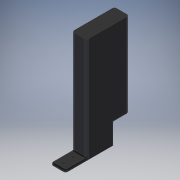
# Autodesk Inventor part: ButtonMountLegs
Saved by Autodesk Inventor 2018 (Build 220112000, 112)
## iProperties
Created: 2018-05-19
Part Number: ButtonMountLegs
Material: Generic
Document SubType Name: Modeling
Designer: reide
Density: 1 g/cm^3
Appearance: Default
Author: reide
Autodesk Inventor part; units mm, degrees
(part 1 of 2)
ref_plane "YZ Plane" through (0, 0, 0) normal (1, 0, 0) x (0, 1, 0)
sketch "Sketch1" plane through (0, 0, 0) normal (0, 0, 1) x (1, 0, 0)
  circle A0 centre (68.6105, -28.321) radius 1.63 projected
  arc A1 (92.5111, 275.0837) -> (88.5111, 275.0837) centre (90.5111, 275.0837) ccw projected
  line L0 (92.5111, 275.0837) -> (92.5111, 230.0837) projected
  arc A2 (88.5111, 230.0837) -> (92.5111, 230.0837) centre (90.5111, 230.0837) ccw projected
  line L1 (88.5111, 230.0837) -> (88.5111, 275.0837) projected
  arc A3 (47.5111, 275.0837) -> (43.5111, 275.0837) centre (45.5111, 275.0837) ccw projected
  line L2 (47.5111, 275.0837) -> (47.5111, 230.0837) projected
  arc A4 (43.5111, 230.0837) -> (47.5111, 230.0837) centre (45.5111, 230.0837) ccw projected
  line L3 (43.5111, 230.0837) -> (43.5111, 275.0837) projected
  circle A5 centre (6.132, -79.3472) radius 1.25 projected
  circle A6 centre (145.3842, 185.8247) radius 1.5 projected
  circle A7 centre (153.8932, -1.3222) radius 1.5 projected
  circle A8 centre (145.3842, -79.3472) radius 1.5 projected
  circle A9 centre (129.8902, 6.8528) radius 1.5 projected
  circle A10 centre (116.3012, -71.1722) radius 1.5 projected
  circle A11 centre (129.8902, 272.0247) radius 1.5 projected
  circle A12 centre (129.8902, 185.8247) radius 1.5 projected
  circle A13 centre (116.3012, 263.8497) radius 1.5 projected
  circle A14 centre (-17.871, -71.1722) radius 1.5 projected
  circle A15 centre (6.132, 6.8528) radius 1.5 projected
  circle A16 centre (19.721, -1.3222) radius 1.5 projected
  circle A17 centre (-17.871, 263.8497) radius 1.5 projected
  circle A18 centre (-9.362, 272.0247) radius 1.5 projected
  circle A19 centre (-9.362, 185.8247) radius 1.5 projected
  circle A20 centre (19.721, 193.9997) radius 1.5 projected
  circle A21 centre (19.721, 263.8497) radius 1.5 projected
  circle A22 centre (6.132, 185.8247) radius 1.5 projected
  circle A23 centre (6.132, 272.0247) radius 1.5 projected
  circle A24 centre (-17.871, 193.9997) radius 1.5 projected
  circle A25 centre (19.721, -71.1722) radius 1.5 projected
  circle A26 centre (-9.362, -79.3472) radius 1.5 projected
  circle A27 centre (-9.362, 6.8528) radius 1.5 projected
  circle A28 centre (-17.871, -1.3222) radius 1.5 projected
  circle A29 centre (116.3012, 193.9997) radius 1.5 projected
  circle A30 centre (153.8932, 193.9997) radius 1.5 projected
  circle A31 centre (153.8932, 263.8497) radius 1.5 projected
  circle A32 centre (145.3842, 6.8528) radius 1.5 projected
  circle A33 centre (129.8902, -79.3472) radius 1.5 projected
  circle A34 centre (153.8932, -71.1722) radius 1.5 projected
  circle A35 centre (116.3012, -1.3222) radius 1.5 projected
  circle A36 centre (145.3842, 272.0247) radius 1.5 projected
  arc A37 (-56.4499, 266.1206) -> (-81.2372, 206.8201) centre (44.5185, 189.0856) ccw projected
  arc A38 (-81.2372, 206.8201) -> (-81.2372, -14.1426) centre (702.1899, 96.3387) ccw projected
  arc A39 (-81.2372, -14.1426) -> (-56.4499, -73.4431) centre (44.5185, 3.5918) ccw projected
  ellipse E0 centre (68.0111, 96.3387) end of major axis (68.0111, -141.4053) minor radius 177.8 (-56.4499, -73.4431) -> (192.4721, -73.4431) ccw projected
  arc A40 (192.4721, -73.4431) -> (217.2594, -14.1426) centre (91.5037, 3.5918) ccw projected
  arc A41 (217.2594, -14.1426) -> (217.2594, 206.8201) centre (-566.1677, 96.3387) ccw projected
  arc A42 (217.2594, 206.8201) -> (192.4721, 266.1206) centre (91.5037, 189.0856) ccw projected
  ellipse E1 centre (68.0111, 96.3387) end of major axis (68.0111, -141.4053) minor radius 177.8 (192.4721, 266.1206) -> (-56.4499, 266.1206) ccw projected
  line L4 (127.3658, 171.3576) -> (131.3658, 171.3576) projected
  arc A43 (131.3658, 168.3578) -> (131.3658, 171.3576) centre (131.3658, 169.8577) ccw projected
  line L5 (131.3658, 168.3578) -> (127.3658, 168.3578) projected
  arc A44 (127.3658, 171.3576) -> (127.3658, 168.3578) centre (127.3658, 169.8577) ccw projected
  line L6 (127.3198, 106.6744) -> (131.3198, 106.6744) projected
  arc A45 (131.3198, 103.6746) -> (131.3198, 106.6744) centre (131.3198, 105.1745) ccw projected
  line L7 (131.3198, 103.6746) -> (127.3198, 103.6746) projected
  arc A46 (127.3198, 106.6744) -> (127.3198, 103.6746) centre (127.3198, 105.1745) ccw projected
  line L8 (12.8629, 171.439) -> (16.8629, 171.439) projected
  arc A47 (16.8629, 168.4391) -> (16.8629, 171.439) centre (16.8629, 169.9391) ccw projected
  line L9 (16.8629, 168.4391) -> (12.8629, 168.4391) projected
  arc A48 (12.8629, 171.439) -> (12.8629, 168.4391) centre (12.8629, 169.9391) ccw projected
  line L10 (12.8169, 106.6744) -> (16.8169, 106.6744) projected
  arc A49 (16.8169, 103.6746) -> (16.8169, 106.6744) centre (16.8169, 105.1745) ccw projected
  line L11 (16.8169, 103.6746) -> (12.8169, 103.6746) projected
  arc A50 (12.8169, 106.6744) -> (12.8169, 103.6746) centre (12.8169, 105.1745) ccw projected
  arc A51 (101.8543, 86.6033) -> (98.8567, 86.6032) centre (100.3555, 86.6032) ccw projected
  line L12 (101.8543, 86.6033) -> (101.8544, 82.6033) projected
  arc A52 (98.8565, 82.6033) -> (101.8544, 82.6033) centre (100.3555, 82.6032) ccw projected
  line L13 (98.8565, 82.6033) -> (98.8567, 86.6032) projected
  arc A53 (101.9362, 200.9947) -> (98.9379, 201.0395) centre (100.4367, 200.9934) ccw projected
  line L14 (101.9362, 200.9947) -> (101.9357, 196.9932) projected
  arc A54 (98.9377, 196.9935) -> (101.9357, 196.9932) centre (100.4367, 196.9934) ccw projected
  line L15 (98.9377, 196.9935) -> (98.9379, 201.0395) projected
  line L16 (34.0863, 189.3896) -> (34.0865, 193.3895) projected
  arc A55 (37.0841, 193.3896) -> (34.0865, 193.3895) centre (35.5853, 193.3895) ccw projected
  line L17 (37.0841, 193.3896) -> (37.0843, 189.3896) projected
  arc A56 (34.0863, 189.3896) -> (37.0843, 189.3896) centre (35.5853, 189.3895) ccw projected
  arc A57 (101.8488, 78.9533) -> (98.8512, 78.9533) centre (100.35, 78.9533) ccw projected
  line L18 (101.8488, 78.9533) -> (101.849, 74.9533) projected
  arc A58 (98.851, 74.9533) -> (101.849, 74.9533) centre (100.35, 74.9533) ccw projected
  line L19 (98.851, 74.9533) -> (98.8512, 78.9533) projected
  circle A59 centre (95.163, 40.4375) radius 1.25 projected
  circle A60 centre (46.141, 40.2217) radius 1.25 projected
  circle A61 centre (36.616, 12.9421) radius 1.25 projected
  circle A62 centre (36.616, -11.1741) radius 1.25 projected
  circle A63 centre (46.141, -14.3491) radius 1.25 projected
  circle A64 centre (36.616, 37.0467) radius 1.25 projected
  circle A65 centre (95.163, -4.4165) radius 1.25 projected
  arc A66 (101.9301, 193.3866) -> (98.9325, 193.3865) centre (100.4313, 193.3865) ccw projected
  line L20 (101.9301, 193.3866) -> (101.9303, 189.3866) projected
  arc A67 (98.9323, 189.3866) -> (101.9303, 189.3866) centre (100.4313, 189.3865) ccw projected
  line L21 (98.9323, 189.3866) -> (98.9325, 193.3865) projected
  arc A68 (37.0788, 78.9992) -> (34.0812, 78.9993) centre (35.58, 78.9992) ccw projected
  line L22 (37.0788, 78.9992) -> (37.079, 74.9993) projected
  arc A69 (34.081, 74.9993) -> (37.079, 74.9993) centre (35.58, 74.9992) ccw projected
  line L23 (34.081, 74.9993) -> (34.0812, 78.9993) projected
  arc A70 (37.0841, 201.0395) -> (34.0865, 201.0395) centre (35.5853, 201.0395) ccw projected
  line L24 (37.0841, 201.0395) -> (37.0843, 197.0395) projected
  arc A71 (34.0863, 197.0396) -> (37.0843, 197.0395) centre (35.5853, 197.0395) ccw projected
  line L25 (34.0863, 197.0396) -> (34.0865, 201.0395) projected
  arc A72 (37.0792, 86.6494) -> (34.0816, 86.6493) centre (35.5804, 86.6492) ccw projected
  line L26 (37.0792, 86.6494) -> (37.0794, 82.6493) projected
  arc A73 (34.0814, 82.6493) -> (37.0794, 82.6493) centre (35.5804, 82.6492) ccw projected
  line L27 (34.0814, 82.6493) -> (34.0816, 86.6493) projected
  line L28 (9.1669, 103.6742) -> (5.1669, 103.6742) projected
  arc A74 (5.1669, 106.6741) -> (5.1669, 103.6742) centre (5.1669, 105.1742) ccw projected
  line L29 (5.1669, 106.6741) -> (9.1669, 106.6741) projected
  arc A75 (9.1669, 103.6742) -> (9.1669, 106.6741) centre (9.1669, 105.1742) ccw projected
  line L30 (5.1669, 171.4444) -> (9.1669, 171.4444) projected
  arc A76 (9.1669, 168.4446) -> (9.1669, 171.4444) centre (9.1669, 169.9445) ccw projected
  line L31 (9.1669, 168.4446) -> (5.1669, 168.4446) projected
  arc A77 (5.1669, 171.4444) -> (5.1669, 168.4446) centre (5.1669, 169.9445) ccw projected
  line L32 (119.6698, 106.6744) -> (123.6698, 106.6744) projected
  arc A78 (123.6698, 103.6746) -> (123.6698, 106.6744) centre (123.6698, 105.1745) ccw projected
  line L33 (123.6698, 103.6746) -> (119.6698, 103.6746) projected
  arc A79 (119.6698, 106.6744) -> (119.6698, 103.6746) centre (119.6698, 105.1745) ccw projected
  line L34 (119.7158, 171.3631) -> (123.7158, 171.3631) projected
  arc A80 (123.7158, 168.3632) -> (123.7158, 171.3631) centre (123.7158, 169.8631) ccw projected
  line L35 (123.7158, 168.3632) -> (119.7158, 168.3632) projected
  arc A81 (119.7158, 171.3631) -> (119.7158, 168.3632) centre (119.7158, 169.8631) ccw projected
  circle A82 centre (68.0111, 137.616) radius 35 projected
  line L36 (82.971, 43.3967) -> (82.971, -17.5241) projected
  line L37 (82.971, -17.5241) -> (52.491, -17.5241) projected
  line L38 (52.491, -17.5241) -> (52.491, 43.3967) projected
  line L39 (52.491, 43.3967) -> (82.971, 43.3967) projected
  circle A83 centre (56.9111, -110.4053) radius 1.5 projected
  circle A84 centre (79.1111, -110.4053) radius 1.5 projected
  circle A85 centre (77.2861, -128.5803) radius 1.5 projected
  circle A86 centre (85.0931, -46.904) radius 1.5 projected
  circle A87 centre (92.2681, -54.079) radius 1.5 projected
  circle A88 centre (53.9141, -54.079) radius 1.5 projected
  circle A89 centre (61.0891, -46.904) radius 1.5 projected
  circle A90 centre (58.7361, -128.5803) radius 1.5 projected
  circle A91 centre (79.1111, -118.4053) radius 1.5 projected
  circle A92 centre (56.9111, -118.4053) radius 1.5 projected
  circle A93 centre (35.6216, 318.7587) radius 1.25 projected
  circle A94 centre (100.4006, 248.9087) radius 1.25 projected
  circle A95 centre (100.4006, 318.7587) radius 1.25 projected
  circle A96 centre (35.6216, 248.9087) radius 1.25 projected
  line L40 (68.0111, 137.616) -> (68.0111, -141.4053)
  line L41 (68.0111, -141.4053) -> (68.0111, 334.0827)
  line L42 (68.0111, 96.3387) -> (-88.9891, 96.3387)
  line L43 (16.9653, 102.9185) -> (4.9653, 102.9185) projected
  arc A97 (4.9653, 118.4285) -> (3.9653, 117.4285) centre (4.9653, 117.4285) ccw projected
  line L44 (4.9653, 118.4285) -> (16.9653, 118.4285) projected
  arc A98 (17.9653, 117.4285) -> (16.9653, 118.4285) centre (16.9653, 117.4285) ccw projected
  line L45 (17.9653, 117.4285) -> (17.9653, 102.9185) projected
  arc A99 (16.9653, 101.9185) -> (17.9653, 102.9185) centre (16.9653, 102.9185) ccw projected
  line L46 (16.9653, 101.9185) -> (4.9653, 101.9185) projected
  arc A100 (3.9653, 102.9185) -> (4.9653, 101.9185) centre (4.9653, 102.9185) ccw projected
  line L47 (3.9653, 117.4285) -> (3.9653, 102.9185) projected
  circle A101 centre (7.1403, 105.0935) radius 1.5 projected
  circle A102 centre (14.7903, 105.0935) radius 1.5 projected
  line L48 (17.6724, 96.3387) -> (3.9653, 96.3387)
  line L49 (3.9653, 96.3387) -> (3.9653, 101.9185)
  line L50 (3.9653, 101.9185) -> (17.6724, 101.9185)
  line L51 (17.6724, 101.9185) -> (17.6724, 96.3387)
  line L52 (17.6724, 96.3387) -> (3.9653, 96.3387)
  line L53 (3.9653, 96.3387) -> (3.9653, 56.3387)
  line L54 (3.9653, 56.3387) -> (17.6724, 56.3387)
  line L55 (17.6724, 56.3387) -> (17.6724, 96.3387)
  circle A103 centre (125.2036, 96.9184) radius 1.75 projected
  circle A104 centre (10.8185, 96.9184) radius 1.75 projected
  circle A105 centre (10.8187, 86.9184) radius 1.75 projected
  circle A106 centre (125.2035, 86.9184) radius 1.75 projected
  circle A107 centre (125.2039, 71.3387) radius 1.75 projected
  circle A108 centre (10.8188, 71.3387) radius 1.75 projected
  circle A109 centre (10.8188, 61.3387) radius 1.75 projected
  circle A110 centre (125.2039, 61.3387) radius 1.75 projected
  point P0 (0, 0)
  dimension "d0" = 40
  constraints: 22 end point, 4 parallel, 2 horizontal, 2 perpendicular, 1 point on circle, 1 point on line, 1 vertical, 4 other
  measures "d0" distance of L54.end L48.start
ref_plane "Work Plane1" through (4.9653, 102.9185, 2) normal (0, 0, 1) x (1, 0, 0)
extrude "Extrusion1" add sketch "Sketch1" along normal up to surface (2 mm away) contours L55 L54 L53 L42 A104 | L42 A104 L49 L50 L46 L51 | A104 L42 | L42 A104 | A105 | A108 | A109
sketch "Sketch2" plane through (3.9653, 101.9185, 2) normal (0, 0, 1) x (1, 0, 0)
  line L0 (13.7071, -45.5798) -> (13.7071, 0) projected
  line L1 (13.7071, -45.5798) -> (13.7071, 34.4202)
  line L2 (0, -45.5798) -> (13.7071, -45.5798) projected
  line L3 (0, -45.5798) -> (0, -5.5798)
  line L4 (0, 0) -> (0, -45.5798) projected
  line L5 (0, -5.5798) -> (0, -25.5798)
  line L6 (0, -25.5798) -> (13.7071, -25.5798)
  line L7 (13.7071, -25.5798) -> (0, -25.5798)
  line L8 (0, -25.5798) -> (0, 0)
  line L9 (0, 0) -> (13.7071, 0)
  line L10 (13.7071, 0) -> (13.7071, -25.5798)
  circle A0 centre (64.6452, -130.2395) radius 1.63 projected
  arc A1 (88.5458, 173.1652) -> (84.5458, 173.1652) centre (86.5458, 173.1652) ccw projected
  line L11 (88.5458, 173.1652) -> (88.5458, 128.1652) projected
  arc A2 (84.5458, 128.1652) -> (88.5458, 128.1652) centre (86.5458, 128.1652) ccw projected
  line L12 (84.5458, 128.1652) -> (84.5458, 173.1652) projected
  arc A3 (43.5458, 173.1652) -> (39.5458, 173.1652) centre (41.5458, 173.1652) ccw projected
  line L13 (43.5458, 173.1652) -> (43.5458, 128.1652) projected
  arc A4 (39.5458, 128.1652) -> (43.5458, 128.1652) centre (41.5458, 128.1652) ccw projected
  line L14 (39.5458, 128.1652) -> (39.5458, 173.1652) projected
  circle A5 centre (2.1667, -181.2657) radius 1.25 projected
  circle A6 centre (141.4189, 83.9062) radius 1.5 projected
  circle A7 centre (149.9279, -103.2407) radius 1.5 projected
  circle A8 centre (141.4189, -181.2657) radius 1.5 projected
  circle A9 centre (125.9249, -95.0657) radius 1.5 projected
  circle A10 centre (112.3359, -173.0907) radius 1.5 projected
  circle A11 centre (125.9249, 170.1062) radius 1.5 projected
  circle A12 centre (125.9249, 83.9062) radius 1.5 projected
  circle A13 centre (112.3359, 161.9312) radius 1.5 projected
  circle A14 centre (-21.8363, -173.0907) radius 1.5 projected
  circle A15 centre (2.1667, -95.0657) radius 1.5 projected
  circle A16 centre (15.7557, -103.2407) radius 1.5 projected
  circle A17 centre (-21.8363, 161.9312) radius 1.5 projected
  circle A18 centre (-13.3273, 170.1062) radius 1.5 projected
  circle A19 centre (-13.3273, 83.9062) radius 1.5 projected
  circle A20 centre (15.7557, 92.0812) radius 1.5 projected
  circle A21 centre (15.7557, 161.9312) radius 1.5 projected
  circle A22 centre (2.1667, 83.9062) radius 1.5 projected
  circle A23 centre (2.1667, 170.1062) radius 1.5 projected
  circle A24 centre (-21.8363, 92.0812) radius 1.5 projected
  circle A25 centre (15.7557, -173.0907) radius 1.5 projected
  circle A26 centre (-13.3273, -181.2657) radius 1.5 projected
  circle A27 centre (-13.3273, -95.0657) radius 1.5 projected
  circle A28 centre (-21.8363, -103.2407) radius 1.5 projected
  circle A29 centre (112.3359, 92.0812) radius 1.5 projected
  circle A30 centre (149.9279, 92.0812) radius 1.5 projected
  circle A31 centre (149.9279, 161.9312) radius 1.5 projected
  circle A32 centre (141.4189, -95.0657) radius 1.5 projected
  circle A33 centre (125.9249, -181.2657) radius 1.5 projected
  circle A34 centre (149.9279, -173.0907) radius 1.5 projected
  circle A35 centre (112.3359, -103.2407) radius 1.5 projected
  circle A36 centre (141.4189, 170.1062) radius 1.5 projected
  arc A37 (-60.4152, 164.2021) -> (-85.2025, 104.9016) centre (40.5532, 87.1671) ccw projected
  arc A38 (-85.2025, 104.9016) -> (-85.2025, -116.0611) centre (698.2246, -5.5798) ccw projected
  arc A39 (-85.2025, -116.0611) -> (-60.4152, -175.3616) centre (40.5532, -98.3267) ccw projected
  ellipse E0 centre (64.0458, -5.5798) end of major axis (64.0458, -243.3238) minor radius 177.8 (-60.4152, -175.3616) -> (188.5068, -175.3616) ccw projected
  arc A40 (188.5068, -175.3616) -> (213.2941, -116.0611) centre (87.5384, -98.3267) ccw projected
  arc A41 (213.2941, -116.0611) -> (213.2941, 104.9016) centre (-570.133, -5.5798) ccw projected
  arc A42 (213.2941, 104.9016) -> (188.5068, 164.2021) centre (87.5384, 87.1671) ccw projected
  ellipse E1 centre (64.0458, -5.5798) end of major axis (64.0458, -243.3238) minor radius 177.8 (188.5068, 164.2021) -> (-60.4152, 164.2021) ccw projected
  line L15 (123.4005, 69.4391) -> (127.4005, 69.4391) projected
  arc A43 (127.4005, 66.4393) -> (127.4005, 69.4391) centre (127.4005, 67.9392) ccw projected
  line L16 (127.4005, 66.4393) -> (123.4005, 66.4393) projected
  arc A44 (123.4005, 69.4391) -> (123.4005, 66.4393) centre (123.4005, 67.9392) ccw projected
  line L17 (123.3545, 4.7559) -> (127.3545, 4.7559) projected
  arc A45 (127.3545, 1.7561) -> (127.3545, 4.7559) centre (127.3545, 3.256) ccw projected
  line L18 (127.3545, 1.7561) -> (123.3545, 1.7561) projected
  arc A46 (123.3545, 4.7559) -> (123.3545, 1.7561) centre (123.3545, 3.256) ccw projected
  line L19 (8.8976, 69.5205) -> (12.8976, 69.5205) projected
  arc A47 (12.8976, 66.5206) -> (12.8976, 69.5205) centre (12.8976, 68.0206) ccw projected
  line L20 (12.8976, 66.5206) -> (8.8976, 66.5206) projected
  arc A48 (8.8976, 69.5205) -> (8.8976, 66.5206) centre (8.8976, 68.0206) ccw projected
  line L21 (8.8516, 4.7559) -> (12.8516, 4.7559) projected
  arc A49 (12.8516, 1.7561) -> (12.8516, 4.7559) centre (12.8516, 3.256) ccw projected
  line L22 (12.8516, 1.7561) -> (8.8516, 1.7561) projected
  arc A50 (8.8516, 4.7559) -> (8.8516, 1.7561) centre (8.8516, 3.256) ccw projected
  arc A51 (97.889, -15.3152) -> (94.8914, -15.3153) centre (96.3902, -15.3153) ccw projected
  line L23 (97.889, -15.3152) -> (97.8892, -19.3152) projected
  arc A52 (94.8912, -19.3152) -> (97.8892, -19.3152) centre (96.3902, -19.3153) ccw projected
  line L24 (94.8912, -19.3152) -> (94.8914, -15.3153) projected
  arc A53 (97.9709, 99.0762) -> (94.9726, 99.121) centre (96.4714, 99.0749) ccw projected
  line L25 (97.9709, 99.0762) -> (97.9704, 95.0747) projected
  arc A54 (94.9724, 95.075) -> (97.9704, 95.0747) centre (96.4714, 95.0749) ccw projected
  line L26 (94.9724, 95.075) -> (94.9726, 99.121) projected
  line L27 (30.121, 87.4711) -> (30.1212, 91.471) projected
  arc A55 (33.1188, 91.4711) -> (30.1212, 91.471) centre (31.62, 91.471) ccw projected
  line L28 (33.1188, 91.4711) -> (33.119, 87.4711) projected
  arc A56 (30.121, 87.4711) -> (33.119, 87.4711) centre (31.62, 87.471) ccw projected
  arc A57 (97.8835, -22.9652) -> (94.8859, -22.9652) centre (96.3847, -22.9652) ccw projected
  line L29 (97.8835, -22.9652) -> (97.8837, -26.9652) projected
  arc A58 (94.8858, -26.9652) -> (97.8837, -26.9652) centre (96.3847, -26.9652) ccw projected
  line L30 (94.8858, -26.9652) -> (94.8859, -22.9652) projected
  circle A59 centre (91.1977, -61.481) radius 1.25 projected
  circle A60 centre (42.1757, -61.6968) radius 1.25 projected
  circle A61 centre (32.6507, -88.9764) radius 1.25 projected
  circle A62 centre (32.6507, -113.0926) radius 1.25 projected
  circle A63 centre (42.1757, -116.2676) radius 1.25 projected
  circle A64 centre (32.6507, -64.8718) radius 1.25 projected
  circle A65 centre (91.1977, -106.335) radius 1.25 projected
  arc A66 (97.9648, 91.4681) -> (94.9672, 91.468) centre (96.466, 91.468) ccw projected
  line L31 (97.9648, 91.4681) -> (97.965, 87.4681) projected
  arc A67 (94.967, 87.4681) -> (97.965, 87.4681) centre (96.466, 87.468) ccw projected
  line L32 (94.967, 87.4681) -> (94.9672, 91.468) projected
  arc A68 (33.1136, -22.9193) -> (30.116, -22.9192) centre (31.6148, -22.9193) ccw projected
  line L33 (33.1136, -22.9193) -> (33.1137, -26.9192) projected
  arc A69 (30.1158, -26.9192) -> (33.1137, -26.9192) centre (31.6148, -26.9193) ccw projected
  line L34 (30.1158, -26.9192) -> (30.116, -22.9192) projected
  arc A70 (33.1188, 99.121) -> (30.1212, 99.121) centre (31.62, 99.121) ccw projected
  line L35 (33.1188, 99.121) -> (33.119, 95.121) projected
  arc A71 (30.121, 95.1211) -> (33.119, 95.121) centre (31.62, 95.121) ccw projected
  line L36 (30.121, 95.1211) -> (30.1212, 99.121) projected
  arc A72 (33.1139, -15.2691) -> (30.1163, -15.2692) centre (31.6151, -15.2693) ccw projected
  line L37 (33.1139, -15.2691) -> (33.1141, -19.2692) projected
  arc A73 (30.1161, -19.2692) -> (33.1141, -19.2692) centre (31.6151, -19.2693) ccw projected
  line L38 (30.1161, -19.2692) -> (30.1163, -15.2692) projected
  line L39 (5.2016, 1.7558) -> (1.2016, 1.7558) projected
  arc A74 (1.2016, 4.7556) -> (1.2016, 1.7558) centre (1.2016, 3.2557) ccw projected
  line L40 (1.2016, 4.7556) -> (5.2016, 4.7556) projected
  arc A75 (5.2016, 1.7558) -> (5.2016, 4.7556) centre (5.2016, 3.2557) ccw projected
  line L41 (1.2016, 69.5259) -> (5.2016, 69.5259) projected
  arc A76 (5.2016, 66.5261) -> (5.2016, 69.5259) centre (5.2016, 68.026) ccw projected
  line L42 (5.2016, 66.5261) -> (1.2016, 66.5261) projected
  arc A77 (1.2016, 69.5259) -> (1.2016, 66.5261) centre (1.2016, 68.026) ccw projected
  line L43 (115.7045, 4.7559) -> (119.7045, 4.7559) projected
  arc A78 (119.7045, 1.7561) -> (119.7045, 4.7559) centre (119.7045, 3.256) ccw projected
  line L44 (119.7045, 1.7561) -> (115.7045, 1.7561) projected
  arc A79 (115.7045, 4.7559) -> (115.7045, 1.7561) centre (115.7045, 3.256) ccw projected
  line L45 (115.7505, 69.4446) -> (119.7505, 69.4446) projected
  arc A80 (119.7505, 66.4447) -> (119.7505, 69.4446) centre (119.7505, 67.9446) ccw projected
  line L46 (119.7505, 66.4447) -> (115.7505, 66.4447) projected
  arc A81 (115.7505, 69.4446) -> (115.7505, 66.4447) centre (115.7505, 67.9446) ccw projected
  circle A82 centre (64.0458, 35.6975) radius 35 projected
  line L47 (79.0057, -58.5218) -> (79.0057, -119.4426) projected
  line L48 (79.0057, -119.4426) -> (48.5257, -119.4426) projected
  line L49 (48.5257, -119.4426) -> (48.5257, -58.5218) projected
  line L50 (48.5257, -58.5218) -> (79.0057, -58.5218) projected
  circle A83 centre (52.9458, -212.3238) radius 1.5 projected
  circle A84 centre (75.1458, -212.3238) radius 1.5 projected
  circle A85 centre (73.3208, -230.4988) radius 1.5 projected
  circle A86 centre (81.1278, -148.8225) radius 1.5 projected
  circle A87 centre (88.3028, -155.9975) radius 1.5 projected
  circle A88 centre (49.9488, -155.9975) radius 1.5 projected
  circle A89 centre (57.1238, -148.8225) radius 1.5 projected
  circle A90 centre (54.7708, -230.4988) radius 1.5 projected
  circle A91 centre (75.1458, -220.3238) radius 1.5 projected
  circle A92 centre (52.9458, -220.3238) radius 1.5 projected
  circle A93 centre (31.6563, 216.8402) radius 1.25 projected
  circle A94 centre (96.4353, 146.9902) radius 1.25 projected
  circle A95 centre (96.4353, 216.8402) radius 1.25 projected
  circle A96 centre (31.6563, 146.9902) radius 1.25 projected
  line L51 (64.0458, 35.6975) -> (64.0458, -5.5798)
  circle A97 centre (121.2384, -5.0001) radius 1.75 projected
  circle A98 centre (6.8533, -5.0001) radius 1.75 projected
  circle A99 centre (6.8534, -15.0001) radius 1.75 projected
  circle A100 centre (121.2382, -15.0001) radius 1.75 projected
  circle A101 centre (121.2387, -30.5798) radius 1.75 projected
  circle A102 centre (6.8536, -30.5798) radius 1.75 projected
  circle A103 centre (6.8536, -40.5798) radius 1.75 projected
  circle A104 centre (121.2387, -40.5798) radius 1.75 projected
  point P0 (-3.9653, -101.9185)
  dimension "d3" = 80
  dimension "d4" = 40
  dimension "d5" = 20
  constraints: 18 end point, 3 point on line, 2 parallel, 2 perpendicular, 1 collinear, 1 horizontal, 1 vertical, 2 other
  measures "d3" distance of L0.start L1.end
  measures "d4" distance of L2.start L3.end
  measures "d5" distance of L3.end L5.end
ref_plane "Work Plane2" through (4.9653, 109.2685, 19.05) normal (0, 0, 1) x (1, 0, 0)
extrude "Extrusion2" add sketch "Sketch2" along normal up to surface (17.05 mm away) contours L6 L3 L4 L9 L0 | A98 | A99
sketch "Sketch3" plane through (3.9653, 101.9185, 19.05) normal (0, 0, 1) x (1, 0, 0)
  line L0 (0, -45.5798) -> (0, -25.5798) projected
  line L1 (13.7071, -45.5798) -> (0, -45.5798) projected
  line L2 (13.7071, -25.5798) -> (13.7071, -45.5798) projected
  line L3 (0, 0) -> (13.7071, 0) projected
  line L4 (0, -25.5798) -> (0, 0) projected
  line L5 (13.7071, -25.5798) -> (0, -25.5798) projected
  line L6 (13.7071, 0) -> (13.7071, -25.5798) projected
  line L7 (0, -45.5798) -> (13.7071, -45.5798) projected
  line L8 (0, -45.5798) -> (-80, -45.5798)
  line L9 (0, 0) -> (0, -45.5798) projected
  line L10 (0, -45.5798) -> (0, 34.4202)
  line L11 (13.7071, -45.5798) -> (13.7071, -5.5798)
  line L12 (13.7071, -45.5798) -> (13.7071, 0) projected
  line L13 (13.7071, -5.5798) -> (13.7071, 14.4202)
  line L14 (13.7071, 14.4202) -> (0, 14.4202)
  line L15 (0, 14.4202) -> (0, -25.5798)
  line L16 (0, -25.5798) -> (13.7071, -25.5798)
  line L17 (13.7071, -25.5798) -> (13.7071, 14.4202)
  circle A0 centre (64.6452, -130.2395) radius 1.63 projected
  arc A1 (88.5458, 173.1652) -> (84.5458, 173.1652) centre (86.5458, 173.1652) ccw projected
  line L18 (88.5458, 173.1652) -> (88.5458, 128.1652) projected
  arc A2 (84.5458, 128.1652) -> (88.5458, 128.1652) centre (86.5458, 128.1652) ccw projected
  line L19 (84.5458, 128.1652) -> (84.5458, 173.1652) projected
  arc A3 (43.5458, 173.1652) -> (39.5458, 173.1652) centre (41.5458, 173.1652) ccw projected
  line L20 (43.5458, 173.1652) -> (43.5458, 128.1652) projected
  arc A4 (39.5458, 128.1652) -> (43.5458, 128.1652) centre (41.5458, 128.1652) ccw projected
  line L21 (39.5458, 128.1652) -> (39.5458, 173.1652) projected
  circle A5 centre (2.1667, -181.2657) radius 1.25 projected
  circle A6 centre (141.4189, 83.9062) radius 1.5 projected
  circle A7 centre (149.9279, -103.2407) radius 1.5 projected
  circle A8 centre (141.4189, -181.2657) radius 1.5 projected
  circle A9 centre (125.9249, -95.0657) radius 1.5 projected
  circle A10 centre (112.3359, -173.0907) radius 1.5 projected
  circle A11 centre (125.9249, 170.1062) radius 1.5 projected
  circle A12 centre (125.9249, 83.9062) radius 1.5 projected
  circle A13 centre (112.3359, 161.9312) radius 1.5 projected
  circle A14 centre (-21.8363, -173.0907) radius 1.5 projected
  circle A15 centre (2.1667, -95.0657) radius 1.5 projected
  circle A16 centre (15.7557, -103.2407) radius 1.5 projected
  circle A17 centre (-21.8363, 161.9312) radius 1.5 projected
  circle A18 centre (-13.3273, 170.1062) radius 1.5 projected
  circle A19 centre (-13.3273, 83.9062) radius 1.5 projected
  circle A20 centre (15.7557, 92.0812) radius 1.5 projected
  circle A21 centre (15.7557, 161.9312) radius 1.5 projected
  circle A22 centre (2.1667, 83.9062) radius 1.5 projected
  circle A23 centre (2.1667, 170.1062) radius 1.5 projected
  circle A24 centre (-21.8363, 92.0812) radius 1.5 projected
  circle A25 centre (15.7557, -173.0907) radius 1.5 projected
  circle A26 centre (-13.3273, -181.2657) radius 1.5 projected
  circle A27 centre (-13.3273, -95.0657) radius 1.5 projected
  circle A28 centre (-21.8363, -103.2407) radius 1.5 projected
  circle A29 centre (112.3359, 92.0812) radius 1.5 projected
  circle A30 centre (149.9279, 92.0812) radius 1.5 projected
  circle A31 centre (149.9279, 161.9312) radius 1.5 projected
  circle A32 centre (141.4189, -95.0657) radius 1.5 projected
  circle A33 centre (125.9249, -181.2657) radius 1.5 projected
  circle A34 centre (149.9279, -173.0907) radius 1.5 projected
  circle A35 centre (112.3359, -103.2407) radius 1.5 projected
  circle A36 centre (141.4189, 170.1062) radius 1.5 projected
  arc A37 (-60.4152, 164.2021) -> (-85.2025, 104.9016) centre (40.5532, 87.1671) ccw projected
  arc A38 (-85.2025, 104.9016) -> (-85.2025, -116.0611) centre (698.2246, -5.5798) ccw projected
  arc A39 (-85.2025, -116.0611) -> (-60.4152, -175.3616) centre (40.5532, -98.3267) ccw projected
  ellipse E0 centre (64.0458, -5.5798) end of major axis (64.0458, -243.3238) minor radius 177.8 (-60.4152, -175.3616) -> (188.5068, -175.3616) ccw projected
  arc A40 (188.5068, -175.3616) -> (213.2941, -116.0611) centre (87.5384, -98.3267) ccw projected
  arc A41 (213.2941, -116.0611) -> (213.2941, 104.9016) centre (-570.133, -5.5798) ccw projected
  arc A42 (213.2941, 104.9016) -> (188.5068, 164.2021) centre (87.5384, 87.1671) ccw projected
  ellipse E1 centre (64.0458, -5.5798) end of major axis (64.0458, -243.3238) minor radius 177.8 (188.5068, 164.2021) -> (-60.4152, 164.2021) ccw projected
  line L22 (123.4005, 69.4391) -> (127.4005, 69.4391) projected
  arc A43 (127.4005, 66.4393) -> (127.4005, 69.4391) centre (127.4005, 67.9392) ccw projected
  line L23 (127.4005, 66.4393) -> (123.4005, 66.4393) projected
  arc A44 (123.4005, 69.4391) -> (123.4005, 66.4393) centre (123.4005, 67.9392) ccw projected
  line L24 (123.3545, 4.7559) -> (127.3545, 4.7559) projected
  arc A45 (127.3545, 1.7561) -> (127.3545, 4.7559) centre (127.3545, 3.256) ccw projected
  line L25 (127.3545, 1.7561) -> (123.3545, 1.7561) projected
  arc A46 (123.3545, 4.7559) -> (123.3545, 1.7561) centre (123.3545, 3.256) ccw projected
  line L26 (8.8976, 69.5205) -> (12.8976, 69.5205) projected
  arc A47 (12.8976, 66.5206) -> (12.8976, 69.5205) centre (12.8976, 68.0206) ccw projected
  line L27 (12.8976, 66.5206) -> (8.8976, 66.5206) projected
  arc A48 (8.8976, 69.5205) -> (8.8976, 66.5206) centre (8.8976, 68.0206) ccw projected
  line L28 (8.8516, 4.7559) -> (12.8516, 4.7559) projected
  arc A49 (12.8516, 1.7561) -> (12.8516, 4.7559) centre (12.8516, 3.256) ccw projected
  line L29 (12.8516, 1.7561) -> (8.8516, 1.7561) projected
  arc A50 (8.8516, 4.7559) -> (8.8516, 1.7561) centre (8.8516, 3.256) ccw projected
  arc A51 (97.889, -15.3152) -> (94.8914, -15.3153) centre (96.3902, -15.3153) ccw projected
  line L30 (97.889, -15.3152) -> (97.8892, -19.3152) projected
  arc A52 (94.8912, -19.3152) -> (97.8892, -19.3152) centre (96.3902, -19.3153) ccw projected
  line L31 (94.8912, -19.3152) -> (94.8914, -15.3153) projected
  arc A53 (97.9709, 99.0762) -> (94.9726, 99.121) centre (96.4714, 99.0749) ccw projected
  line L32 (97.9709, 99.0762) -> (97.9704, 95.0747) projected
  arc A54 (94.9724, 95.075) -> (97.9704, 95.0747) centre (96.4714, 95.0749) ccw projected
  line L33 (94.9724, 95.075) -> (94.9726, 99.121) projected
  line L34 (30.121, 87.4711) -> (30.1212, 91.471) projected
  arc A55 (33.1188, 91.4711) -> (30.1212, 91.471) centre (31.62, 91.471) ccw projected
  line L35 (33.1188, 91.4711) -> (33.119, 87.4711) projected
  arc A56 (30.121, 87.4711) -> (33.119, 87.4711) centre (31.62, 87.471) ccw projected
  arc A57 (97.8835, -22.9652) -> (94.8859, -22.9652) centre (96.3847, -22.9652) ccw projected
  line L36 (97.8835, -22.9652) -> (97.8837, -26.9652) projected
  arc A58 (94.8858, -26.9652) -> (97.8837, -26.9652) centre (96.3847, -26.9652) ccw projected
  line L37 (94.8858, -26.9652) -> (94.8859, -22.9652) projected
  circle A59 centre (91.1977, -61.481) radius 1.25 projected
  circle A60 centre (42.1757, -61.6968) radius 1.25 projected
  circle A61 centre (32.6507, -88.9764) radius 1.25 projected
  circle A62 centre (32.6507, -113.0926) radius 1.25 projected
  circle A63 centre (42.1757, -116.2676) radius 1.25 projected
  circle A64 centre (32.6507, -64.8718) radius 1.25 projected
  circle A65 centre (91.1977, -106.335) radius 1.25 projected
  arc A66 (97.9648, 91.4681) -> (94.9672, 91.468) centre (96.466, 91.468) ccw projected
  line L38 (97.9648, 91.4681) -> (97.965, 87.4681) projected
  arc A67 (94.967, 87.4681) -> (97.965, 87.4681) centre (96.466, 87.468) ccw projected
  line L39 (94.967, 87.4681) -> (94.9672, 91.468) projected
  arc A68 (33.1136, -22.9193) -> (30.116, -22.9192) centre (31.6148, -22.9193) ccw projected
  line L40 (33.1136, -22.9193) -> (33.1137, -26.9192) projected
  arc A69 (30.1158, -26.9192) -> (33.1137, -26.9192) centre (31.6148, -26.9193) ccw projected
  line L41 (30.1158, -26.9192) -> (30.116, -22.9192) projected
  arc A70 (33.1188, 99.121) -> (30.1212, 99.121) centre (31.62, 99.121) ccw projected
  line L42 (33.1188, 99.121) -> (33.119, 95.121) projected
  arc A71 (30.121, 95.1211) -> (33.119, 95.121) centre (31.62, 95.121) ccw projected
  line L43 (30.121, 95.1211) -> (30.1212, 99.121) projected
  arc A72 (33.1139, -15.2691) -> (30.1163, -15.2692) centre (31.6151, -15.2693) ccw projected
  line L44 (33.1139, -15.2691) -> (33.1141, -19.2692) projected
  arc A73 (30.1161, -19.2692) -> (33.1141, -19.2692) centre (31.6151, -19.2693) ccw projected
  line L45 (30.1161, -19.2692) -> (30.1163, -15.2692) projected
  line L46 (5.2016, 1.7558) -> (1.2016, 1.7558) projected
  arc A74 (1.2016, 4.7556) -> (1.2016, 1.7558) centre (1.2016, 3.2557) ccw projected
  line L47 (1.2016, 4.7556) -> (5.2016, 4.7556) projected
  arc A75 (5.2016, 1.7558) -> (5.2016, 4.7556) centre (5.2016, 3.2557) ccw projected
  line L48 (1.2016, 69.5259) -> (5.2016, 69.5259) projected
  arc A76 (5.2016, 66.5261) -> (5.2016, 69.5259) centre (5.2016, 68.026) ccw projected
  line L49 (5.2016, 66.5261) -> (1.2016, 66.5261) projected
  arc A77 (1.2016, 69.5259) -> (1.2016, 66.5261) centre (1.2016, 68.026) ccw projected
  line L50 (115.7045, 4.7559) -> (119.7045, 4.7559) projected
  arc A78 (119.7045, 1.7561) -> (119.7045, 4.7559) centre (119.7045, 3.256) ccw projected
  line L51 (119.7045, 1.7561) -> (115.7045, 1.7561) projected
  arc A79 (115.7045, 4.7559) -> (115.7045, 1.7561) centre (115.7045, 3.256) ccw projected
  line L52 (115.7505, 69.4446) -> (119.7505, 69.4446) projected
  arc A80 (119.7505, 66.4447) -> (119.7505, 69.4446) centre (119.7505, 67.9446) ccw projected
  line L53 (119.7505, 66.4447) -> (115.7505, 66.4447) projected
  arc A81 (115.7505, 69.4446) -> (115.7505, 66.4447) centre (115.7505, 67.9446) ccw projected
  circle A82 centre (64.0458, 35.6975) radius 35 projected
  line L54 (79.0057, -58.5218) -> (79.0057, -119.4426) projected
  line L55 (79.0057, -119.4426) -> (48.5257, -119.4426) projected
  line L56 (48.5257, -119.4426) -> (48.5257, -58.5218) projected
  line L57 (48.5257, -58.5218) -> (79.0057, -58.5218) projected
  circle A83 centre (52.9458, -212.3238) radius 1.5 projected
  circle A84 centre (75.1458, -212.3238) radius 1.5 projected
  circle A85 centre (73.3208, -230.4988) radius 1.5 projected
  circle A86 centre (81.1278, -148.8225) radius 1.5 projected
  circle A87 centre (88.3028, -155.9975) radius 1.5 projected
  circle A88 centre (49.9488, -155.9975) radius 1.5 projected
  circle A89 centre (57.1238, -148.8225) radius 1.5 projected
  circle A90 centre (54.7708, -230.4988) radius 1.5 projected
  circle A91 centre (75.1458, -220.3238) radius 1.5 projected
  circle A92 centre (52.9458, -220.3238) radius 1.5 projected
  circle A93 centre (31.6563, 216.8402) radius 1.25 projected
  circle A94 centre (96.4353, 146.9902) radius 1.25 projected
  circle A95 centre (96.4353, 216.8402) radius 1.25 projected
  circle A96 centre (31.6563, 146.9902) radius 1.25 projected
  line L58 (64.0458, 35.6975) -> (64.0458, -5.5798)
  line L59 (13.7071, -25.5798) -> (0, -25.5798) projected
  circle A97 centre (121.2384, -5.0001) radius 1.75 projected
  circle A98 centre (6.8533, -5.0001) radius 1.75 projected
  circle A99 centre (6.8534, -15.0001) radius 1.75 projected
  circle A100 centre (121.2382, -15.0001) radius 1.75 projected
  point P0 (-3.9653, -101.9185)
  dimension "d8" = 80
  dimension "d9" = 80
  dimension "d10" = 40
  dimension "d11" = 20
  constraints: 18 end point, 2 collinear, 2 parallel, 2 point on line, 1 horizontal, 1 perpendicular, 1 vertical, 2 other
  measures "d8" distance of L0.start L8.end
  measures "d9" distance of L0.start L10.end
  measures "d10" distance of L1.start L11.end
  measures "d11" distance of L11.end L13.end
extrude "Extrusion3" add sketch "Sketch3" along normal blind 80 contours L4 L3 L6 L5 | L10 A74 L46 A75 L47 L14 L13 A49 L28 A50 L29 L3 | L10 A74 L47 A75 L46 | A49 L29 A50 L28 L13 | A98 | A99
sketch "Sketch5" plane through (3.9653, 56.3387, 2) normal (0, 0, 1) x (1, 0, 0)
  line L0 (0, 0) -> (0, 20) projected
  line L1 (13.7071, 0) -> (0, 0) projected
  line L2 (13.7071, 20) -> (13.7071, 0) projected
  line L3 (128.0916, 20) -> (114.3845, 20) projected
  line L4 (114.3845, 0) -> (114.3845, 20) projected
  line L5 (128.0916, 0) -> (114.3845, 0) projected
  line L6 (128.0916, 20) -> (128.0916, 0) projected
  line L7 (0, 0) -> (13.7071, 0) projected
  line L8 (6.8536, 0) -> (6.8536, 5)
  circle A0 centre (6.8536, 5) radius 1.5
  line L9 (13.7071, 20) -> (0, 20) projected
  line L10 (6.8536, 20) -> (6.8536, 15)
  circle A1 centre (6.8536, 15) radius 1.5
  circle A2 centre (64.6452, -84.6598) radius 1.63 projected
  arc A3 (88.5458, 218.745) -> (84.5458, 218.745) centre (86.5458, 218.745) ccw projected
  line L11 (88.5458, 218.745) -> (88.5458, 173.745) projected
  arc A4 (84.5458, 173.745) -> (88.5458, 173.745) centre (86.5458, 173.745) ccw projected
  line L12 (84.5458, 173.745) -> (84.5458, 218.745) projected
  arc A5 (43.5458, 218.745) -> (39.5458, 218.745) centre (41.5458, 218.745) ccw projected
  line L13 (43.5458, 218.745) -> (43.5458, 173.745) projected
  arc A6 (39.5458, 173.745) -> (43.5458, 173.745) centre (41.5458, 173.745) ccw projected
  line L14 (39.5458, 173.745) -> (39.5458, 218.745) projected
  circle A7 centre (2.1667, -135.686) radius 1.25 projected
  circle A8 centre (141.4189, 129.486) radius 1.5 projected
  circle A9 centre (149.9279, -57.661) radius 1.5 projected
  circle A10 centre (141.4189, -135.686) radius 1.5 projected
  circle A11 centre (125.9249, -49.486) radius 1.5 projected
  circle A12 centre (112.3359, -127.511) radius 1.5 projected
  circle A13 centre (125.9249, 215.686) radius 1.5 projected
  circle A14 centre (125.9249, 129.486) radius 1.5 projected
  circle A15 centre (112.3359, 207.511) radius 1.5 projected
  circle A16 centre (-21.8363, -127.511) radius 1.5 projected
  circle A17 centre (2.1667, -49.486) radius 1.5 projected
  circle A18 centre (15.7557, -57.661) radius 1.5 projected
  circle A19 centre (-21.8363, 207.511) radius 1.5 projected
  circle A20 centre (-13.3273, 215.686) radius 1.5 projected
  circle A21 centre (-13.3273, 129.486) radius 1.5 projected
  circle A22 centre (15.7557, 137.661) radius 1.5 projected
  circle A23 centre (15.7557, 207.511) radius 1.5 projected
  circle A24 centre (2.1667, 129.486) radius 1.5 projected
  circle A25 centre (2.1667, 215.686) radius 1.5 projected
  circle A26 centre (-21.8363, 137.661) radius 1.5 projected
  circle A27 centre (15.7557, -127.511) radius 1.5 projected
  circle A28 centre (-13.3273, -135.686) radius 1.5 projected
  circle A29 centre (-13.3273, -49.486) radius 1.5 projected
  circle A30 centre (-21.8363, -57.661) radius 1.5 projected
  circle A31 centre (112.3359, 137.661) radius 1.5 projected
  circle A32 centre (149.9279, 137.661) radius 1.5 projected
  circle A33 centre (149.9279, 207.511) radius 1.5 projected
  circle A34 centre (141.4189, -49.486) radius 1.5 projected
  circle A35 centre (125.9249, -135.686) radius 1.5 projected
  circle A36 centre (149.9279, -127.511) radius 1.5 projected
  circle A37 centre (112.3359, -57.661) radius 1.5 projected
  circle A38 centre (141.4189, 215.686) radius 1.5 projected
  arc A39 (-60.4152, 209.7818) -> (-85.2025, 150.4814) centre (40.5532, 132.7469) ccw projected
  arc A40 (-85.2025, 150.4814) -> (-85.2025, -70.4814) centre (698.2246, 40) ccw projected
  arc A41 (-85.2025, -70.4814) -> (-60.4152, -129.7818) centre (40.5532, -52.7469) ccw projected
  ellipse E0 centre (64.0458, 40) end of major axis (64.0458, -197.744) minor radius 177.8 (-60.4152, -129.7818) -> (188.5068, -129.7818) ccw projected
  arc A42 (188.5068, -129.7818) -> (213.2941, -70.4814) centre (87.5384, -52.7469) ccw projected
  arc A43 (213.2941, -70.4814) -> (213.2941, 150.4814) centre (-570.133, 40) ccw projected
  arc A44 (213.2941, 150.4814) -> (188.5068, 209.7818) centre (87.5384, 132.7469) ccw projected
  ellipse E1 centre (64.0458, 40) end of major axis (64.0458, -197.744) minor radius 177.8 (188.5068, 209.7818) -> (-60.4152, 209.7818) ccw projected
  line L15 (123.4005, 115.0189) -> (127.4005, 115.0189) projected
  arc A45 (127.4005, 112.0191) -> (127.4005, 115.0189) centre (127.4005, 113.519) ccw projected
  line L16 (127.4005, 112.0191) -> (123.4005, 112.0191) projected
  arc A46 (123.4005, 115.0189) -> (123.4005, 112.0191) centre (123.4005, 113.519) ccw projected
  line L17 (123.3545, 50.3357) -> (127.3545, 50.3357) projected
  arc A47 (127.3545, 47.3359) -> (127.3545, 50.3357) centre (127.3545, 48.8358) ccw projected
  line L18 (127.3545, 47.3359) -> (123.3545, 47.3359) projected
  arc A48 (123.3545, 50.3357) -> (123.3545, 47.3359) centre (123.3545, 48.8358) ccw projected
  line L19 (8.8976, 115.1002) -> (12.8976, 115.1002) projected
  arc A49 (12.8976, 112.1004) -> (12.8976, 115.1002) centre (12.8976, 113.6003) ccw projected
  line L20 (12.8976, 112.1004) -> (8.8976, 112.1004) projected
  arc A50 (8.8976, 115.1002) -> (8.8976, 112.1004) centre (8.8976, 113.6003) ccw projected
  line L21 (8.8516, 50.3357) -> (12.8516, 50.3357) projected
  arc A51 (12.8516, 47.3359) -> (12.8516, 50.3357) centre (12.8516, 48.8358) ccw projected
  line L22 (12.8516, 47.3359) -> (8.8516, 47.3359) projected
  arc A52 (8.8516, 50.3357) -> (8.8516, 47.3359) centre (8.8516, 48.8358) ccw projected
  arc A53 (97.889, 30.2646) -> (94.8914, 30.2645) centre (96.3902, 30.2645) ccw projected
  line L23 (97.889, 30.2646) -> (97.8892, 26.2646) projected
  arc A54 (94.8912, 26.2646) -> (97.8892, 26.2646) centre (96.3902, 26.2645) ccw projected
  line L24 (94.8912, 26.2646) -> (94.8914, 30.2645) projected
  arc A55 (97.9709, 144.656) -> (94.9726, 144.7008) centre (96.4714, 144.6547) ccw projected
  line L25 (97.9709, 144.656) -> (97.9704, 140.6545) projected
  arc A56 (94.9724, 140.6548) -> (97.9704, 140.6545) centre (96.4714, 140.6547) ccw projected
  line L26 (94.9724, 140.6548) -> (94.9726, 144.7008) projected
  line L27 (30.121, 133.0508) -> (30.1212, 137.0507) projected
  arc A57 (33.1188, 137.0509) -> (30.1212, 137.0507) centre (31.62, 137.0508) ccw projected
  line L28 (33.1188, 137.0509) -> (33.119, 133.0509) projected
  arc A58 (30.121, 133.0508) -> (33.119, 133.0509) centre (31.62, 133.0508) ccw projected
  arc A59 (97.8835, 22.6145) -> (94.8859, 22.6146) centre (96.3847, 22.6145) ccw projected
  line L29 (97.8835, 22.6145) -> (97.8837, 18.6146) projected
  arc A60 (94.8858, 18.6146) -> (97.8837, 18.6146) centre (96.3847, 18.6145) ccw projected
  line L30 (94.8858, 18.6146) -> (94.8859, 22.6146) projected
  circle A61 centre (91.1977, -15.9012) radius 1.25 projected
  circle A62 centre (42.1757, -16.117) radius 1.25 projected
  circle A63 centre (32.6507, -43.3966) radius 1.25 projected
  circle A64 centre (32.6507, -67.5128) radius 1.25 projected
  circle A65 centre (42.1757, -70.6878) radius 1.25 projected
  circle A66 centre (32.6507, -19.292) radius 1.25 projected
  circle A67 centre (91.1977, -60.7552) radius 1.25 projected
  arc A68 (97.9648, 137.0479) -> (94.9672, 137.0478) centre (96.466, 137.0478) ccw projected
  line L31 (97.9648, 137.0479) -> (97.965, 133.0479) projected
  arc A69 (94.967, 133.0479) -> (97.965, 133.0479) centre (96.466, 133.0478) ccw projected
  line L32 (94.967, 133.0479) -> (94.9672, 137.0478) projected
  arc A70 (33.1136, 22.6605) -> (30.116, 22.6605) centre (31.6148, 22.6605) ccw projected
  line L33 (33.1136, 22.6605) -> (33.1137, 18.6606) projected
  arc A71 (30.1158, 18.6606) -> (33.1137, 18.6606) centre (31.6148, 18.6605) ccw projected
  line L34 (30.1158, 18.6606) -> (30.116, 22.6605) projected
  arc A72 (33.1188, 144.7008) -> (30.1212, 144.7007) centre (31.62, 144.7007) ccw projected
  line L35 (33.1188, 144.7008) -> (33.119, 140.7008) projected
  arc A73 (30.121, 140.7008) -> (33.119, 140.7008) centre (31.62, 140.7007) ccw projected
  line L36 (30.121, 140.7008) -> (30.1212, 144.7007) projected
  arc A74 (33.1139, 30.3106) -> (30.1163, 30.3106) centre (31.6151, 30.3105) ccw projected
  line L37 (33.1139, 30.3106) -> (33.1141, 26.3106) projected
  arc A75 (30.1161, 26.3106) -> (33.1141, 26.3106) centre (31.6151, 26.3105) ccw projected
  line L38 (30.1161, 26.3106) -> (30.1163, 30.3106) projected
  line L39 (5.2016, 47.3355) -> (1.2016, 47.3355) projected
  arc A76 (1.2016, 50.3354) -> (1.2016, 47.3355) centre (1.2016, 48.8354) ccw projected
  line L40 (1.2016, 50.3354) -> (5.2016, 50.3354) projected
  arc A77 (5.2016, 47.3355) -> (5.2016, 50.3354) centre (5.2016, 48.8354) ccw projected
  line L41 (1.2016, 115.1057) -> (5.2016, 115.1057) projected
  arc A78 (5.2016, 112.1058) -> (5.2016, 115.1057) centre (5.2016, 113.6058) ccw projected
  line L42 (5.2016, 112.1058) -> (1.2016, 112.1058) projected
  arc A79 (1.2016, 115.1057) -> (1.2016, 112.1058) centre (1.2016, 113.6058) ccw projected
  line L43 (115.7045, 50.3357) -> (119.7045, 50.3357) projected
  arc A80 (119.7045, 47.3359) -> (119.7045, 50.3357) centre (119.7045, 48.8358) ccw projected
  line L44 (119.7045, 47.3359) -> (115.7045, 47.3359) projected
  arc A81 (115.7045, 50.3357) -> (115.7045, 47.3359) centre (115.7045, 48.8358) ccw projected
  line L45 (115.7505, 115.0243) -> (119.7505, 115.0243) projected
  arc A82 (119.7505, 112.0245) -> (119.7505, 115.0243) centre (119.7505, 113.5244) ccw projected
  line L46 (119.7505, 112.0245) -> (115.7505, 112.0245) projected
  arc A83 (115.7505, 115.0243) -> (115.7505, 112.0245) centre (115.7505, 113.5244) ccw projected
  circle A84 centre (64.0458, 81.2773) radius 35 projected
  line L47 (79.0057, -12.942) -> (79.0057, -73.8628) projected
  line L48 (79.0057, -73.8628) -> (48.5257, -73.8628) projected
  line L49 (48.5257, -73.8628) -> (48.5257, -12.942) projected
  line L50 (48.5257, -12.942) -> (79.0057, -12.942) projected
  circle A85 centre (52.9458, -166.744) radius 1.5 projected
  circle A86 centre (75.1458, -166.744) radius 1.5 projected
  circle A87 centre (73.3208, -184.919) radius 1.5 projected
  circle A88 centre (81.1278, -103.2427) radius 1.5 projected
  circle A89 centre (88.3028, -110.4177) radius 1.5 projected
  circle A90 centre (49.9488, -110.4177) radius 1.5 projected
  circle A91 centre (57.1238, -103.2427) radius 1.5 projected
  circle A92 centre (54.7708, -184.919) radius 1.5 projected
  circle A93 centre (75.1458, -174.744) radius 1.5 projected
  circle A94 centre (52.9458, -174.744) radius 1.5 projected
  circle A95 centre (31.6563, 262.42) radius 1.25 projected
  circle A96 centre (96.4353, 192.57) radius 1.25 projected
  circle A97 centre (96.4353, 262.42) radius 1.25 projected
  circle A98 centre (31.6563, 192.57) radius 1.25 projected
  line L51 (64.0458, 81.2773) -> (64.0458, 40)
  line L52 (114.3845, 20) -> (128.0916, 20)
  line L53 (128.0916, 0) -> (128.0916, 20)
  line L54 (114.3845, 0) -> (128.0916, 0)
  line L55 (114.3845, 20) -> (114.3845, 0)
  line L56 (128.0916, 0) -> (114.3845, 0)
  line L57 (121.2381, 0) -> (121.2381, 5)
  circle A99 centre (121.2381, 5) radius 1.5
  line L58 (114.3845, 20) -> (128.0916, 20)
  line L59 (121.2381, 20) -> (121.2381, 15)
  circle A100 centre (121.2381, 15) radius 1.5
  line L60 (13.7071, 20) -> (0, 20) projected
  circle A101 centre (121.2384, 40.5797) radius 1.75 projected
  circle A102 centre (6.8533, 40.5797) radius 1.75 projected
  circle A103 centre (6.8534, 30.5797) radius 1.75 projected
  circle A104 centre (121.2382, 30.5797) radius 1.75 projected
  circle A105 centre (121.2387, 15) radius 1.75 projected
  circle A106 centre (6.8536, 15) radius 1.75 projected
  circle A107 centre (6.8536, 5) radius 1.75 projected
  circle A108 centre (121.2387, 5) radius 1.75 projected
  point P0 (-3.9653, -56.3387)
  dimension "d15" = 5
  dimension "d16" = 3
  dimension "d17" = 5
  dimension "d18" = 3
  constraints: 22 end point, 6 symmetric about line, 4 centre point, 4 coincident, 3 vertical, 2 midpoint, 4 other
  measures "d15" distance of L8.start L8.end
  measures "d16" diameter of A0
  measures "d17" distance of L10.start L10.end
  measures "d18" diameter of A1
extrude "Extrusion4" cut sketch "Sketch5" against normal blind 50 contours A0 | A1 | A99 | A100
fillet "Fillet1" radius 2 6 edges at (3.9653, 56.3387, 1) (17.6724, 56.3387, 1) (3.9653, 116.3387, 59.05) (17.6724, 116.3387, 59.05) (17.6724, 76.3387, 50.525) (3.9653, 76.3387, 50.525)
fillet "Fillet2" radius 1 9 edges at (4.5511, 56.9245, 2) (10.8188, 56.3387, 2) (17.0866, 56.9245, 2) (17.6724, 67.3387, 2) (17.6724, 77.3387, 2) (3.9653, 77.3387, 2) (3.9653, 67.3387, 2) (17.6724, 101.9185, 9.525) (3.9653, 101.9185, 9.525)
fillet "Fillet3" radius 1 7 edges at (17.0866, 115.7529, 19.05) (10.8188, 116.3387, 19.05) (4.5511, 115.7529, 19.05) (3.9653, 101.4185, 19.05) (3.9653, 108.1286, 19.05) (17.6724, 101.4185, 19.05) (17.6724, 108.1286, 19.05)
fillet "Fillet4" radius 1 3 edges at (4.1952, 77.4076, 1.638) (17.4424, 77.4076, 1.638) (10.8188, 76.3387, 2)
fillet "Fillet5" radius 1 3 edges at (17.3795, 101.6256, 19.3429) (4.2582, 101.6256, 19.3429) (10.8188, 101.9185, 19.05)